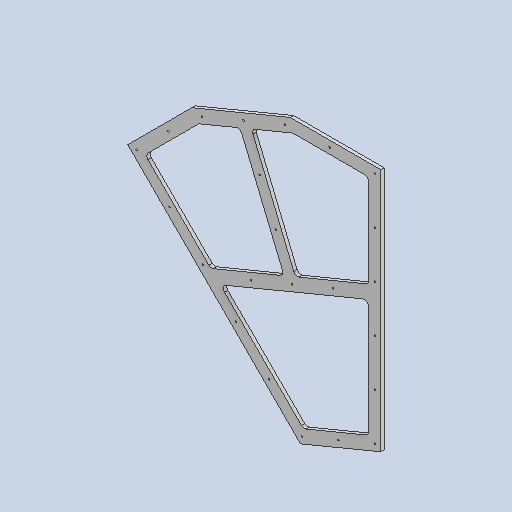
# Autodesk Inventor part: ДМФ 01 56 Крепление сетки к кассете v2.0
Saved by Autodesk Inventor 2025 (Build 290162010, 162A)
## iProperties
Created: 2024-05-05
Part Number: ДМФ 01 56 Крепление сетки к кассете v2.0
Material: Generic
Document SubType Name: Modeling
Designer: pokla
Density: 1 g/cm^3
Appearance: Default
Author: pokla
Autodesk Inventor part; units mm, degrees
ref_plane "YZ Plane" through (0, 0, 0) normal (1, 0, 0) x (0, 1, 0)
ref_plane "XZ Plane" through (0, 0, 0) normal (0, 1, 0) x (-1, 0, 0)
ref_plane "XY Plane" through (0, 0, 0) normal (0, 0, 1) x (1, 0, 0)
sketch "Sketch1" plane through (0, 0, 0) normal (0, 0, 1) x (1, 0, 0)
  line L0 (0, 277.6336) -> (196.3166, 196.3166) construction
  line L1 (196.3166, 196.3166) -> (277.6336, 0) construction
  line L2 (277.6336, 0) -> (196.3166, -196.3166) construction
  line L3 (196.3166, -196.3166) -> (0, -277.6336) construction
  line L4 (0, -277.6336) -> (-196.3166, -196.3166) construction
  line L5 (-196.3166, -196.3166) -> (-277.6336, 0) construction
  line L6 (-277.6336, 0) -> (-196.3166, 196.3166) construction
  line L7 (-196.3166, 196.3166) -> (0, 277.6336)
  line L8 (-196.3166, 196.3166) -> (0, 277.6336)
  line L9 (-461.2666, 773.8898) -> (-221.0579, 873.3874)
  line L10 (-98.1583, 236.9751) -> (-341.1623, 823.6386) construction
  line L11 (-221.0579, 873.3874) -> (0, 873.3874)
  line L12 (0, 873.3874) -> (0, 277.6336)
  line L13 (-461.2666, 773.8898) -> (-617.5782, 617.5782)
  line L14 (-617.5782, 617.5782) -> (-196.3166, 196.3166)
  point P0 (0, 0)
  point P1 (0, 0)
  dimension "d0" = 513
  dimension "d2" = 260
  dimension "d3" = 635
  constraints: 30 end point, 2 midpoint, 1 coincident, 1 horizontal, 1 parallel, 1 perpendicular, 1 symmetric about line, 1 vertical, 1 vertical alignment, 17 other
  measures "d0" distance between parallel lines of L5 L1
  measures "d2" distance of L9.start L9.end
  measures "d3" distance of L10.end L10.start
extrude "Extrusion1" add sketch "Sketch1" along normal mid plane 8
sketch "Sketch2" plane through (0, 0, 4) normal (0, 0, 1) x (1, 0, 0)
  line L0 (-221.0579, 873.3874) -> (-461.2666, 773.8898) projected
  line L1 (-461.2666, 773.8898) -> (-617.5782, 617.5782) projected
  line L2 (-236.3886, 531.4957) -> (-415.0608, 457.4872)
  line L3 (-196.3166, 196.3166) -> (0, 277.6336) projected
  line L4 (-98.1583, 236.9751) -> (-341.1623, 823.6386) construction
  line L5 (-617.5782, 617.5782) -> (-196.3166, 196.3166) projected
  line L6 (-415.0608, 457.4872) -> (-575.1518, 617.5782)
  line L7 (-575.1518, 617.5782) -> (-444.273, 748.457)
  line L8 (-444.273, 748.457) -> (-343.54, 790.182)
  line L9 (-236.3886, 531.4957) -> (-343.54, 790.182)
  line L10 (-208.6722, 542.9762) -> (-30, 616.9847)
  line L11 (-30, 616.9847) -> (-30, 843.3874)
  line L12 (-30, 843.3874) -> (-215.0906, 843.3874)
  line L13 (-215.0906, 843.3874) -> (-315.8236, 801.6625)
  line L14 (-208.6722, 542.9762) -> (-315.8236, 801.6625)
  line L15 (0, 277.6336) -> (0, 873.3874) projected
  line L16 (-415.0608, 457.4872) -> (-30, 616.9847) construction
  line L17 (-392.0998, 434.5262) -> (-30, 584.5129)
  line L18 (-189.2776, 231.704) -> (-30, 297.679)
  line L19 (-30, 297.679) -> (-30, 584.5129)
  line L20 (-189.2776, 231.704) -> (-392.0998, 434.5262)
  point P0 (0, 0)
  dimension "d11" = 30
  dimension "d12" = 280
  dimension "d13" = 30
  dimension "d14" = 30
  dimension "d15" = 15
  dimension "d21" = 30
  dimension "d22" = 30
  dimension "d23" = 30
  dimension "d24" = 30
  constraints: 32 end point, 5 parallel, 5 symmetric about line, 2 midpoint, 1 collinear
  measures "d11" distance between parallel lines of L5 L6
  measures "d12" distance between parallel lines of L8 L2
  measures "d13" distance between parallel lines of L0 L8
  measures "d14" distance between parallel lines of L1 L7
  measures "d15" distance between parallel lines of L9 L4
  measures "d21" distance between parallel lines of L16 L17
  measures "d22" distance between parallel lines of L5 L20
  measures "d23" distance between parallel lines of L19 L15
  measures "d24" distance between parallel lines of L18 L3
extrude "Extrusion2" cut sketch "Sketch2" against normal up to surface (8 mm away)
fillet "Fillet1" radius 10 12 edges at (-575.1518, 617.5782, 0) (-343.54, 790.182, 0) (-236.3886, 531.4957, 0) (-415.0608, 457.4872, 0) (-315.8236, 801.6625, 0) (-30, 843.3874, 0) (-30, 616.9847, 0) (-208.6722, 542.9762, 0) (-392.0998, 434.5262, 0) (-30, 584.5129, 0) (-30, 297.679, 0) (-189.2776, 231.704, 0)
sketch "Sketch5" plane through (0, 0, 4) normal (0, 0, 1) x (1, 0, 0)
  line L0 (-221.0579, 873.3874) -> (-461.2666, 773.8898) projected
  line L1 (0, 873.3874) -> (-221.0579, 873.3874) projected
  line L2 (-461.2666, 773.8898) -> (-617.5782, 617.5782) projected
  line L3 (-617.5782, 617.5782) -> (-196.3166, 196.3166) projected
  line L4 (-196.3166, 196.3166) -> (0, 277.6336) projected
  line L5 (0, 277.6336) -> (0, 873.3874) projected
  line L6 (-15, 858.3874) -> (-218.0743, 858.3874) construction
  line L7 (-218.0743, 858.3874) -> (-452.7698, 761.1734) construction
  line L8 (-452.7698, 761.1734) -> (-596.365, 617.5782) construction
  line L9 (-596.365, 617.5782) -> (-192.7971, 214.0103) construction
  line L10 (-192.7971, 214.0103) -> (-15, 287.6563) construction
  line L11 (-15, 287.6563) -> (-15, 858.3874) construction
  line L12 (-378.273, 440.2535) -> (-43.8268, 578.7856) projected
  line L13 (-212.4991, 552.215) -> (-311.9967, 792.4237) projected
  line L14 (-418.5803, 439.7935) -> (-15, 606.962) construction
  line L15 (-216.7902, 523.3778) -> (-335.422, 809.7804) construction
  circle A0 centre (-335.422, 809.7804) radius 2
  circle A1 centre (-216.7902, 523.3778) radius 2
  circle A2 centre (-295.8793, 714.3159) radius 2
  circle A3 centre (-256.3367, 618.8515) radius 2
  circle A4 centre (-596.365, 617.5782) radius 2
  circle A5 centre (-515.5729, 536.7861) radius 2
  circle A6 centre (-434.7809, 455.9941) radius 2
  circle A7 centre (-353.9889, 375.2021) radius 2
  circle A8 centre (-273.1968, 294.41) radius 2
  circle A9 centre (-192.4048, 213.618) radius 2
  circle A10 centre (-317.0311, 481.8566) radius 2
  circle A11 centre (-103.8986, 250.8333) radius 2
  circle A12 centre (-518.5832, 695.3599) radius 2
  circle A13 centre (-437.0488, 767.6852) radius 2
  circle A14 centre (-15, 858.3874) radius 2
  circle A15 centre (-15, 744.1302) radius 2
  circle A16 centre (-15, 629.873) radius 2
  circle A17 centre (-15, 515.6158) radius 2
  circle A18 centre (-15, 401.3586) radius 2
  circle A19 centre (-15, 287.1014) radius 2
  circle A20 centre (-116.5492, 564.8989) radius 2
  circle A21 centre (-125, 858.3874) radius 2
  circle A22 centre (-233.7953, 851.8756) radius 2
  point P0 (0, 0)
  dimension "d32" = 15
  dimension "d33" = 15
  dimension "d34" = 15
  dimension "d35" = 4
  dimension "d37" = 103.33
  dimension "d38" = 103.33
  dimension "d43" = 114.2572
  dimension "d49" = 108.5
  dimension "d50" = 110
  dimension "d51" = 110
  constraints: 23 centre point, 16 end point, 9 symmetric about line, 8 equal radius, 7 point on line, 3 coincident, 3 midpoint, 2 parallel, 25 other
  measures "d32" distance between parallel lines of L5 L11
  measures "d33" distance between parallel lines of L12 L14
  measures "d34" distance between parallel lines of L13 L15
  measures "d35" diameter of A0
  measures "d37" distance of A2.centre A0.centre
  measures "d38" distance of A3.centre A2.centre
  measures "d43" distance of A4.centre A5.centre
  measures "d49" distance of A1.centre A10.centre
  measures "d50" distance of A12.centre A4.centre
  measures "d51" distance of A13.centre A0.centre
extrude "Extrusion4" cut sketch "Sketch5" against normal up to surface (8 mm away) contours A0 | A1 | A2 | A3 | A4 | A5 | A6 | A7 | A8 | A9 | A10 | A11 | A12 | A13 | A14 | A15 | A16 | A17 | A18 | A19 | A20 | A21 | A22
equation "\"d0\" = Барабан_габарит_по_кассетам"
equation "\"d2\" = Кассета_длина_грани"
equation "\"d3\" = Кассета_высота"
equation "\"d11\" = d13"
equation "\"d14\" = d13"
equation "\"d15\" = 0.5 * d13"
equation "\"d21\" = d13"
equation "\"d22\" = d13"
equation "\"d23\" = d13"
equation "\"d24\" = d13"
equation "\"Барабан_габарит_по_кассетам\" = 513"
equation "\"Кассета_длина_грани\" = 260"
equation "\"Кассета_высота\" = 635"
body "Solid1"
